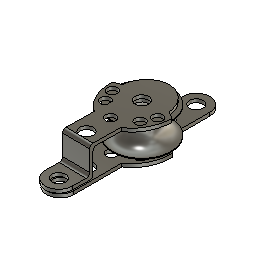
Viadana 8.08 (Autodesk Fusion 360 design; units mm, degrees)
Autodesk Fusion 360 part; units mm, degrees
sketch "Sketch1" plane through (0, 0, 0) normal (0, 0, 1) x (1, 0, 0)
  line L0 (0, 0) -> (0, 48) construction
  circle A0 centre (0, 44) radius 2
  circle A1 centre (0, 4) radius 2
  line L1 (-4, 44) -> (-4, 4)
  line L2 (4, 44) -> (4, 4)
  line L3 (-4, 44) -> (0, 44) construction
  arc A2 (4, 44) -> (-4, 44) centre (0, 44) ccw
  arc A3 (-4, 4) -> (4, 4) centre (0, 4) ccw
  circle A4 centre (0, 28) radius 2
  circle A5 centre (0, 12) radius 2
  ellipse E0 centre (0, 28) end of major axis (0, 17) minor radius 9
  line L4 (0, 39) -> (0, 17)
  line L5 (-9, 28) -> (9, 28)
  ellipse E1 centre (0, 28) end of major axis (7, 28) minor radius 8
  line L6 (-7, 28) -> (7, 28)
  line L7 (0, 20) -> (0, 36)
  spline S0 degree 5 poles (-9, 28) (-8.9919, 28.0122) (-8.9754, 28.0362) (-8.9503, 28.0709) (-8.9116, 28.116) (-8.833, 28.1781) (-8.7018, 28.2534) (-8.504, 28.347) (-8.2469, 28.4567) (-7.9585, 28.5736) (-7.6748, 28.6866) (-7.4315, 28.7857) (-7.2521, 28.8663) (-7.1414, 28.9315) (-7.0654, 29) (-7.006, 29.0815) (-6.9642, 29.1609) (-6.9346, 29.2289) (-6.9157, 29.278) (-6.9065, 29.3035) knots 0 0 0 0 0 0 0.066667 0.133333 0.2 0.266667 0.333333 0.4 0.466667 0.533333 0.6 0.666667 0.733333 0.8 0.866667 0.933333 1 1 1 1 1 1
  line L8 (-7.3689, 28.8) -> (-7.0311, 29)
  line L9 (-9.1, 27.8499) -> (-8.9, 28.1501)
  spline S1 degree 5 poles (9, 28) (8.9919, 28.0122) (8.9754, 28.0362) (8.9503, 28.0709) (8.9116, 28.116) (8.833, 28.1781) (8.7018, 28.2534) (8.504, 28.347) (8.2469, 28.4567) (7.9585, 28.5736) (7.6748, 28.6866) (7.4315, 28.7857) (7.2521, 28.8663) (7.1414, 28.9315) (7.0654, 29) (7.006, 29.0815) (6.9642, 29.1609) (6.9346, 29.2289) (6.9157, 29.278) (6.9065, 29.3035) knots 0 0 0 0 0 0 0.066667 0.133333 0.2 0.266667 0.333333 0.4 0.466667 0.533333 0.6 0.666667 0.733333 0.8 0.866667 0.933333 1 1 1 1 1 1
  line L10 (-7.0215, 28.9866) -> (-6.7914, 29.6204)
  line L11 (9.1, 27.8499) -> (8.9, 28.1501)
  line L12 (7.3689, 28.8) -> (7.0311, 29)
  line L13 (7.0215, 28.9866) -> (6.7914, 29.6204)
  circle A6 centre (0, 19) radius 1.5
  circle A7 centre (6.7777, 26) radius 1.5
  circle A8 centre (-5.1667, 22.5) radius 1.5
  circle A9 centre (-6.7777, 26) radius 1.5
  line L14 (-6.7777, 26) -> (6.7777, 26) construction
  circle A10 centre (5.1667, 22.5) radius 1.5
  line L15 (-5.1667, 22.5) -> (5.1667, 22.5) construction
  circle A11 centre (0, 36) radius 1.5
  point P0 (0, 24)
  point P1 (-8.6, 28.3)
  point P2 (-7.2, 28.9)
  point P3 (7.2, 28.9)
  point P4 (8.6, 28.3)
  point P5 (0, 22.5)
  point P6 (0, 26)
  point P7 (0, 24.5)
  dimension "d3" = 48
  dimension "d4" = 4
  dimension "d5" = 4
  dimension "d6" = 40
  dimension "d7" = 20
  dimension "d8" = 4
  dimension "d9" = 16
  dimension "d10" = 4
  dimension "d11" = 4
  dimension "d12" = 8
  dimension "d15" = 9
  dimension "d16" = 11
  dimension "d17" = 8
  dimension "d18" = 7
  dimension "d19" = 3
  dimension "d20" = 3
  dimension "d21" = 3
  dimension "d23" = 3
  dimension "d24" = 3
  dimension "d25" = 3.5
  dimension "d26" = 3.5
  dimension "d66" = 3
  dimension "d67" = 8
  constraint coincident L0.start origin
  constraint vertical L0
  constraint midpoint L0 P0
  constraint coincident L0 A0.centre
  constraint coincident L0 A1.centre
  constraint parallel L0 L1
  constraint symmetric L0 L1.start L2.start
  constraint symmetric L0 L1.end L2.end
  constraint coincident A0.centre L3.end
  constraint perpendicular L0 L3
  constraint coincident L0.end A2
  constraint coincident L0.start A3
  constraint coincident L0 A4.centre
  constraint coincident L0 A5.centre
  constraint coincident E0 L4.start
  constraint coincident E0 L4.end
  constraint coincident E0 L5.start
  constraint coincident E0 L5.end
  constraint concentric A4 E0
  constraint parallel L0 L4
  constraint coincident E1 L6.start
  constraint coincident E1 L6.end
  constraint coincident E1 L7.start
  constraint coincident E1 L7.end
  constraint concentric A4 E1
  constraint perpendicular L2 L6
  constraint coincident E1 S0.end
  constraint midpoint P2 L8
  constraint midpoint L5.start L9
  constraint midpoint S0.end L10
  constraint symmetric L0 L5.start L5.end
  constraint symmetric L0 P1 P4
  constraint symmetric L0 P2 P3
  constraint symmetric L0 S0.end S1.end
  constraint symmetric L0 L8.start L12.start
  constraint symmetric L0 L8.end L12.end
  constraint symmetric L0 L9.start L11.start
  constraint symmetric L0 L9.end L11.end
  constraint symmetric L0 L10.start L13.start
  constraint symmetric L0 L10.end L13.end
  constraint coincident L4 A6.centre
  constraint coincident A9.centre L14.start
  constraint coincident A7.centre L14.end
  constraint horizontal L14
  constraint coincident A8.centre L15.start
  constraint coincident A10.centre L15.end
  constraint horizontal L15
  constraint midpoint L15 P5
  constraint coincident L7 P5
  constraint midpoint L14 P6
  constraint coincident L0 P7
  constraint coincident A4 P6
  constraint coincident L0 P6
  constraint coincident E1 A7.centre
  constraint coincident L0 L7.end
  measures "d3" distance of L0.start L0.end
  measures "d4" diameter of A0
  measures "d5" diameter of A1
  measures "d6" distance of A0.centre A1.centre
  measures "d7" distance of P0 A0.centre
  measures "d8" distance of L0 L1
  measures "d9" distance of A0.centre A4.centre
  measures "d10" diameter of A4
  measures "d11" diameter of A5
  measures "d12" distance of A1.centre A5.centre
  measures "d15" distance of A4.centre L5.end
  measures "d16" distance of A4.centre L4.end
  measures "d17" distance of A4.centre L7.end
  measures "d18" distance of A4.centre L6.end
  measures "d19" diameter of A9
  measures "d20" diameter of A8
  measures "d21" diameter of A6
  measures "d23" diameter of A7
  measures "d24" diameter of A10
  measures "d25" distance of A6.centre L15
  measures "d26" distance of L14 L15
  measures "d66" diameter of A11
  measures "d67" distance of A0.centre L7.end
extrude "Extrude1" add sketch "Sketch1" along normal blind 1 contours L1 L2 A2 E0 | L1 E0 L4 E1 A11 | L1 A4 L4 L5 E1 L6 L7 A11 | L1 L5 E1 L6 | L2 E0 L4 E1 A11 | L1 E0 L5 E1 A8 A9 | L5 E1 S0 | L1 A4 L4 L5 E1 L6 L7 A6 A8 | L1 L5 E1 L6 A8 A9 | L1 L2 A3 E0 | L1 E0 L4 E1 A6 | L2 L5 E1 L6 | L2 A4 L4 L5 E1 L6 L7 A11 | L2 E0 L5 E1 A7 A10 | L5 E1 S1 | L1 A8 | L1 E1 A8 | L2 E0 L4 E1 A6 | L2 L5 E1 L6 A7 A10 | L2 A4 L4 L5 E1 L6 L7 A6 A10 | L2 E1 A10 picked at (-4.0068, 21.5082) picked at (4.0068, 21.5082) makes body 1
sketch "Sketch1 (2)" plane through (0, 0, 0) normal (0, 1, 0) x (1, 0, 0) in component "roll"
  line L0 (4, 4.25) -> (-4, 4.25)
  line L1 (-4, 4.25) -> (-4, -4.25)
  line L2 (-4, -4.25) -> (4, -4.25)
  line L3 (4, -4.25) -> (4, 4.25)
  line L4 (4, 4.25) -> (-4, -4.25) construction
  line L5 (-4, 4.25) -> (4, -4.25) construction
  circle A0 centre (0, -4.25) radius 3.75
  circle A1 centre (0, 4.25) radius 3.75
  dimension "d27" = 8.5
  dimension "d28" = 8
  dimension "d32" = 7.5
  dimension "d33" = 7.5
  constraint horizontal L0
  constraint perpendicular L0 L1
  constraint parallel L1 L3
  constraint coincident L4 origin
  constraint coincident L5 origin
  constraint midpoint L2 A0.centre
  constraint midpoint L0 A1.centre
  measures "d27" distance of L0.start L2.end
  measures "d28" distance of L0.start L0.end
  measures "d32" diameter of A0
  measures "d33" diameter of A1
revolve "Revolve1" add sketch "Sketch1 (2)" angle 360 about axis through (4, 0, -4.25) along (-1, 0, 0) separate body contours L0 L1 L2 L3 A0 A1 makes body 2 in component "roll"
sketch "Sketch2" plane through (4, 0, 0) normal (1, 0, 0) x (0, 1, 0) in component "roll"
  circle A0 centre (0, -4.25) radius 8.5
  circle A1 centre (0, -4.25) radius 8.5
  circle A2 centre (0, -4.25) radius 2
  dimension "d34" = 4
  constraint concentric A1 A2
  measures "d34" diameter of A2
extrude "Extrude1'" cut sketch "Sketch2" against normal blind 8 contours A2 bodies 2 in component "roll"
sketch "Sketch1 (3)" plane through (0, 0, 0) normal (0, 0, 1) x (1, 0, 0) in component "Plat-up"
  circle A0 centre (5.1667, 22.5) radius 1.5
  circle A1 centre (6.7777, 26) radius 1.5
  circle A2 centre (-6.7777, 26) radius 1.5
  circle A3 centre (0, 19) radius 1.5
  arc A4 (-4, 23.4428) -> (-4, 21.5572) centre (-5.1667, 22.5) ccw
  line L0 (-4, 23.4428) -> (-4, 21.5572)
  circle A5 centre (0, 12) radius 2
  circle A6 centre (0, 28) radius 2
  circle A7 centre (0, 4) radius 2
  circle A8 centre (0, 44) radius 2
  ellipse E0 centre (0, 28) end of major axis (0, 17) minor radius 9 (4, 18.1461) -> (9, 28) ccw
  spline S0 degree 5 poles (9, 28) (8.9919, 28.0122) (8.9754, 28.0362) (8.9503, 28.0709) (8.9116, 28.116) (8.833, 28.1781) (8.7018, 28.2534) (8.504, 28.347) (8.2469, 28.4567) (7.9585, 28.5736) (7.6748, 28.6866) (7.4315, 28.7857) (7.2521, 28.8663) (7.1414, 28.9315) (7.0654, 29) (7.006, 29.0815) (6.9642, 29.1609) (6.9346, 29.2289) (6.9157, 29.278) (6.9065, 29.3035) knots 0 0 0 0 0 0 0.066667 0.133333 0.2 0.266667 0.333333 0.4 0.466667 0.533333 0.6 0.666667 0.733333 0.8 0.866667 0.933333 1 1 1 1 1 1
  ellipse E1 centre (0, 28) end of major axis (0, 36) minor radius 7 (6.9065, 29.3035) -> (4, 34.5652) ccw
  line L1 (4, 34.5652) -> (4, 44)
  arc A9 (4, 44) -> (-4, 44) centre (0, 44) ccw
  line L2 (-4, 44) -> (-4, 34.5652)
  ellipse E2 centre (0, 28) end of major axis (0, 36) minor radius 7 (-4, 34.5652) -> (-6.9065, 29.3035) ccw
  spline S1 degree 5 poles (-6.9065, 29.3035) (-6.9157, 29.278) (-6.9346, 29.2289) (-6.9642, 29.1609) (-7.006, 29.0815) (-7.0654, 29) (-7.1414, 28.9315) (-7.2521, 28.8663) (-7.4315, 28.7857) (-7.6748, 28.6866) (-7.9585, 28.5736) (-8.2469, 28.4567) (-8.504, 28.347) (-8.7018, 28.2534) (-8.833, 28.1781) (-8.9116, 28.116) (-8.9503, 28.0709) (-8.9754, 28.0362) (-8.9919, 28.0122) (-9, 28) knots -1 -1 -1 -1 -1 -1 -0.933333 -0.866667 -0.8 -0.733333 -0.666667 -0.6 -0.533333 -0.466667 -0.4 -0.333333 -0.266667 -0.2 -0.133333 -0.066667 0 0 0 0 0 0
  ellipse E3 centre (0, 28) end of major axis (0, 17) minor radius 9 (-9, 28) -> (-4, 18.1461) ccw
  line L3 (-4, 18.1461) -> (-4, 4)
  arc A10 (-4, 4) -> (4, 4) centre (0, 4) ccw
  line L4 (4, 4) -> (4, 18.1461)
  arc A11 (4, 34.5652) -> (-4, 34.5652) centre (0, 29.7069) ccw
  circle A12 centre (0, 36) radius 1.5
  constraint coincident L1.start A11.start
  constraint coincident L2.end A11.end
extrude "Extrude1''" add sketch "Sketch1 (3)" along normal blind 9 separate body contours E0 S0 E1 E2 S1 E3 L3 A10 L4 A11 A12 | A11 A12 picked at (-0.4609, 35.5317) makes body 3 in component "Plat-up"
ref_plane "WorkPlane1" through (15, 0, 0) normal (1, 0, 0) x (0, 1, 0) in component "Plat-up"
sketch "Sketch2 (2)" plane through (15, 0, 0) normal (1, 0, 0) x (0, 1, 0) in component "Plat-up"
  line L0 (4, 0) -> (0, 0)
  line L1 (4, 0) -> (4, 9)
  line L2 (4, 9) -> (0, 9)
  line L3 (4, 9) -> (4, 0)
  line L4 (4, 0) -> (18.1461, 0)
  line L5 (18.1461, 0) -> (18.1461, 9)
  line L6 (18.1461, 9) -> (4, 9)
  line L7 (4, 9) -> (4, 0)
  line L8 (28, 0) -> (18.1461, 0)
  line L9 (28, 0) -> (28, 9)
  line L10 (28, 9) -> (18.1461, 9)
  line L11 (18.1461, 9) -> (18.1461, 0)
  line L12 (28, 0) -> (29.3035, 0)
  line L13 (29.3035, 0) -> (29.3035, 9)
  line L14 (28, 9) -> (29.3035, 9)
  line L15 (28, 9) -> (28, 0)
  line L16 (34.5652, 0) -> (29.3035, 0)
  line L17 (34.5652, 0) -> (34.5652, 9)
  line L18 (34.5652, 9) -> (29.3035, 9)
  line L19 (29.3035, 9) -> (29.3035, 0)
  line L20 (36, 0) -> (34.5652, 0)
  line L21 (34.5652, 0) -> (34.5652, 9)
  line L22 (36, 9) -> (34.5652, 9)
  line L23 (34.5652, 9) -> (34.5652, 0)
  line L24 (0, 0) -> (36, 0)
  line L25 (36, 9) -> (0, 9)
  line L26 (0, 0) -> (0, 9)
  line L27 (36, 9) -> (36, 0)
  line L28 (10, 8) -> (36, 8)
  line L29 (0, 1) -> (9, 1)
  line L30 (10, 0) -> (10, 8)
  line L31 (9, 1) -> (9, 9)
  dimension "d45" = 1
  dimension "d49" = 9
  dimension "d50" = 1
  dimension "d51" = 1
  constraint coincident L0.end L24.start
  constraint coincident L20.start L24.end
  constraint coincident L22.start L25.start
  constraint coincident L2.end L25.end
  constraint coincident L27 L28.end
  constraint perpendicular L27 L28
  constraint coincident L26 L29.start
  constraint perpendicular L26 L29
  constraint coincident L28 L30.end
  constraint perpendicular L28 L30
  constraint coincident L25 L31.end
  measures "d45" distance of L25 L28
  measures "d49" distance of L29.start L29.end
  measures "d50" distance of L24 L29
  measures "d51" distance of L30 L31
extrude "Extrude2" cut sketch "Sketch2 (2)" against normal blind 32 contours L1 L2 L3 L7 L25 L26 L29 | L1 L3 L6 L7 L25 L29 L31 | L4 L5 L11 L24 L28 L30 | L5 L8 L9 L11 L15 L24 L28 | L9 L12 L13 L15 L19 L24 L28 | L13 L16 L17 L19 L21 L23 L24 L28 | L17 L20 L21 L23 L24 L27 L28 bodies 3 in component "Plat-up"
fillet "Fillet1" radius 1 1 edges at (0, 9, 9) on bodies 3 in component "Plat-up"
fillet "Fillet2" radius 1 1 edges at (0, 9, 1) on bodies 3 in component "Plat-up"
fillet "Fillet3" radius 1 1 edges at (0, 10, 0) on bodies 3 in component "Plat-up"
fillet "Fillet4" radius 1 2 edges at (2, 10, 8) (-2, 10, 8) on bodies 3 in component "Plat-up"
component "roll" placed x (0, 0, -1) y (-0.945428, -0.32583, 0) z (-0.32583, 0.945428, 0) at (-1.3848, 32.0181, 5)
component "Plat1" placed x (1, 0, 0) y (0, 1, 0) z (0, 0, 1) at (0, 0, 0)
component "Plat-up" placed x (0.999852, -0.017176, 0) y (0.017176, 0.999852, 0) z (0, 0, 1) at (-0.4809, 0.0041, 1)
equation "d27 = ( 17 / 2 ) * 1 mm"
